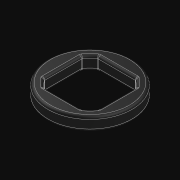
# Autodesk Inventor part: Spacer High Strength
Saved by Autodesk Inventor 2021.3 (Build 253353010, 353A)
## iProperties
Created: 2020-05-16
Part Number: Spacer High Strength
Material: Acetal Resin, Black
Document SubType Name: Modeling
Designer: yuany
Density: 1.425 g/cm^3
Appearance: Smooth - Black
Author: yuany
Autodesk Inventor part; units mm, degrees
ref_plane "YZ Plane" through (0, 0, 0) normal (1, 0, 0) x (0, 1, 0)
ref_plane "XZ Plane" through (0, 0, 0) normal (0, 1, 0) x (-1, 0, 0)
ref_plane "XY Plane" through (0, 0, 0) normal (0, 0, 1) x (1, 0, 0)
sketch "Sketch1" plane through (0, 0, 0) normal (0, 1, 0) x (-1, 0, 0)
  circle A0 centre (0, 0) radius 5
  line L0 (2.2293, 3.2) -> (-2.2293, 3.2)
  line L1 (-3.2, 2.2293) -> (-3.2, -2.2293)
  line L2 (-2.2293, -3.2) -> (2.2293, -3.2)
  line L3 (3.2, -2.2293) -> (3.2, 2.2293)
  arc A1 (3.2, 2.2293) -> (2.2293, 3.2) centre (0, 0) ccw
  arc A2 (2.2293, -3.2) -> (3.2, -2.2293) centre (0, 0) ccw
  arc A3 (-2.2293, 3.2) -> (-3.2, 2.2293) centre (0, 0) ccw
  arc A4 (-3.2, -2.2293) -> (-2.2293, -3.2) centre (0, 0) ccw
  dimension "d0" = 10
  dimension "d2" = 3.2
  dimension "d3" = 3.2
  dimension "d5" = 6.4
  constraints: 8 end point, 8 point on circle, 5 centre point, 2 coincident, 2 parallel, 1 horizontal, 1 perpendicular
  measures "d0" diameter of A0
  measures "d2" distance from line of L0 point (0, 0)
  measures "d3" distance from line of point (0, 0) L3
  measures "d5" distance between parallel lines of L3 L1
extrude "Extrusion1" add sketch "Sketch1" along normal blind 1.5875
fillet "Fillet1" radius 0.3 18 edges at (0, 1.5875, 3.2) (0, 0, 3.2) (-2.7577, 0, 2.7577) (-2.7577, 1.5875, 2.7577) (-3.2, 1.5875, 0) (-3.2, 0, 0) (-2.7577, 0, -2.7577) (0, 0, -3.2) (0, 1.5875, -3.2) (-2.7577, 1.5875, -2.7577) (2.7577, 1.5875, -2.7577) (3.2, 1.5875, 0) (2.7577, 1.5875, 2.7577) (2.7577, 0, -2.7577) (3.2, 0, 0) (2.7577, 0, 2.7577) (5, 0, 0) (5, 1.5875, 0)
fillet "Fillet1" radius 0.1 8 edges at (2.2293, 0.7937, 3.2) (3.2, 0.7937, 2.2293) (3.2, 0.7937, -2.2293) (-3.2, 0.7937, -2.2293) (-2.2293, 0.7937, -3.2) (-3.2, 0.7937, 2.2293) (-2.2293, 0.7937, 3.2) (2.2293, 0.7937, -3.2)
body "Solid1"
